Autodesk Fusion 360 part; units mm, degrees
(part 2 of 2)
  spline S274 degree 3 poles (72.1202, -8.538) (72.5736, -8.6218) (72.8098, -8.637) (73.0288, -8.6009) knots 0 0 0 0 1 1 1 1
extrude "Extrude7" add sketch "Sketch4" along normal blind 0.25 separate body contours S0 S1 S2 S3 S4 S5 S6 S7 S8 S9 S10 S11 S12 S13 S14 S15 S16 S17 S18 S19 S20 S21 S22 L25 L26 S23 S24 S25 S26 S27 S28 S29 S30 | S31 S32 S33 S34 S35 S36 S37 S38 S39 S40 S41 S42 S43 S44 S45 S46 S47 S48 S49 S50 S51 S52 | S167 S168 S169 S170 S171 S172 S173 S174 S175 S176 S177 S178 S179 S180 S181 S182 S183 S184 S185 S186 S187 S188 S189 S190 S191 S192 S193 S194 S195 S196 S197 S198 S199 S200 S201 S202 S203 S204 S205 S206 S207 S208 | S209 S210 S211 S212 S213 S214 S215 S216 S217 S218 S219 S220 S221 S222 S223 S224 S225 S226 S227 S228 S229 S230 S231 L73 L74 L75 L76 S232 S233 S234 S235 S236 S237 S238 S239 S240 S241 S242 S243 S244 S245 S246 S247 S248 S249 S250 S251 S252 S253 S254 S255 S256 S257 S258 S259 S260 S261 S262 S263 S264 L77 L78 L79 L80 S265 S266 S267 S268 S269 S270 S271 S272 S273 S274 makes body 2 at (-71.4286, 5.6913, 5.5) makes body 3 at (-56.3602, 7.5605, 5.5) makes body 4 at (-69.2144, 14.3959, 5.5) makes body 5 at (-63.6424, 15.0623, 5.5)
extrude "Extrude8" add sketch "Sketch4" along normal blind 0.1 separate body contours S53 S54 S55 S56 S57 S58 S59 S60 S61 S62 S63 S64 S65 S66 S67 S68 S69 S70 S71 S72 S73 S74 S75 S76 S77 S78 S79 S80 L27 L28 S81 S82 S83 S84 S85 L29 L30 S86 S87 S88 S89 S90 L31 L32 S91 S92 L33 L34 S93 L35 L36 L37 L38 S94 L39 L40 S95 S96 S97 S98 L41 L42 S99 S100 S101 S102 S103 L43 L44 L45 L46 S104 S105 S106 S107 S108 S109 S110 S111 S112 S113 S114 S115 S116 S117 S118 S119 S120 S121 S122 S123 S124 S125 L47 L48 L49 L50 L51 L52 L53 L54 L55 L56 L57 L58 L59 L60 S126 S127 L61 L62 S128 S129 L63 L64 S130 S131 S132 L65 L66 L67 L68 S133 S134 S135 S136 S137 S138 S139 S140 S141 S142 S143 S144 S145 S146 S147 S148 S149 L69 L70 S150 S151 S152 S153 S154 L71 L72 S155 S156 S157 S158 S159 S160 S161 S162 S163 S164 S165 S166 makes body 6
